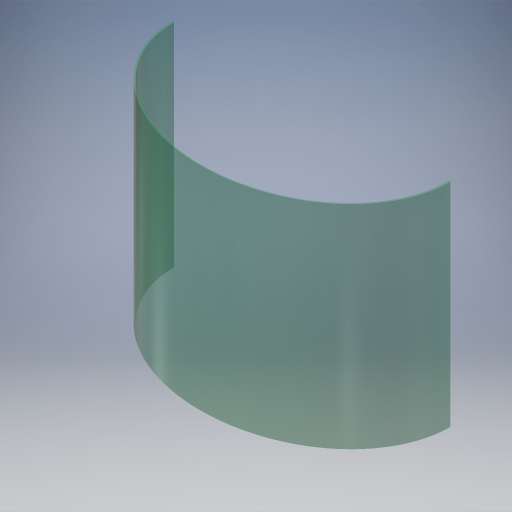
# Autodesk Inventor part: 24_0497_0018
Saved by Autodesk Inventor 2024.3 (Build 283343000, 343)
## iProperties
Created: 2024-05-28
Part Number: 24_0497_0018
Material: LCP-Kunststoff
Document SubType Name: Modeling
Designer: Vogel
Density: 1.626 g/cm^3
Appearance: Klar - Grün 1
Author: Vogel
Autodesk Inventor part; units mm, degrees
ref_plane "YZ Plane" through (0, 0, 0) normal (1, 0, 0) x (0, 1, 0)
ref_plane "XZ Plane" through (0, 0, 0) normal (0, 1, 0) x (-1, 0, 0)
ref_plane "XY Plane" through (0, 0, 0) normal (0, 0, 1) x (1, 0, 0)
sketch "Skizze1" plane through (0, 0, 0) normal (0, 0, 1) x (1, 0, 0)
  line L0 (-212.8, 0) -> (212.8, 0) projected
  line L1 (0, -169.4) -> (0, 169.4) projected
  ellipse E0 centre (0, 0) end of major axis (-150, 0) minor radius 120
  line L2 (0, 120) -> (0, -120) construction
  line L3 (-150, 0) -> (150, 0) construction
  line L4 (0, 0) -> (-152, 0)
  line L5 (0, 0) -> (0, 121)
  ellipse E1 centre (0, 0) end of major axis (0, 121) minor radius 152
  point P0 (152, 0)
  dimension "d0" = 300
  dimension "d1" = 240
  dimension "d34" = 152
  dimension "d35" = 121
  constraints: 8 end point, 6 point on line, 2 coincident, 1 vertical, 10 other
  measures "d0" distance of L3.start L3.end
  measures "d1" distance of L2.start L2.end
  measures "d34" distance from line of L1 L4.end
  measures "d35" distance from line of L5.end L0
extrude "Extrusion3" add sketch "Skizze1" along normal blind 232 contours L0 E0 L1 E1 | L1 E0 L0 E1 picked at (-151.0004, -4.6164) picked at (148.5136, -19.4462)
